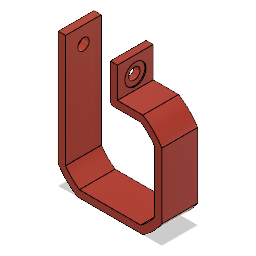
_extruder_mount.6a3fcada-6a02-4eac-834c-371bbe1a886d (Autodesk Fusion 360 design; units mm, degrees)
Autodesk Fusion 360 part; units mm, degrees
sketch "Sketch2" plane through (0, 0, 0) normal (0, 0, 1) x (1, 0, 0)
  line L0 (14.4655, -21) -> (-14.4655, -21)
  line L1 (-21, -14.4655) -> (-21, 14.4655)
  line L2 (1, 21) -> (14.4655, 21)
  line L3 (21, 14.4655) -> (21, -14.4655)
  line L4 (18.0312, -18.0312) -> (-18.0312, 18.0312) construction
  line L5 (-18.0312, -18.0312) -> (18.0312, 18.0312) construction
  arc A0 (21, 14.4655) -> (14.4655, 21) centre (0, 0) ccw
  arc A1 (-21, -14.4655) -> (-14.4655, -21) centre (0, 0) ccw
  arc A2 (14.4655, -21) -> (21, -14.4655) centre (0, 0) ccw
  line L6 (-21, 14.4655) -> (-21, 21)
  line L7 (0.0943, 21.9057) -> (0.0943, 41)
  line L8 (0.0943, 41) -> (-21, 41)
  line L9 (-21, 41) -> (-21, 21)
  line L10 (0.0943, 21.9057) -> (1, 21)
  line L11 (-24.5, 38.866) -> (-24.5, 21)
  line L12 (-24.5, 14.4655) -> (-24.5, 21)
  line L13 (-24.5, -15.5161) -> (-24.5, 14.4655)
  arc A3 (-24.5, -15.5161) -> (-15.5161, -24.5) centre (0, 0) ccw
  line L14 (15.5161, -24.5) -> (-15.5161, -24.5)
  arc A4 (15.5161, -24.5) -> (24.5, -15.5161) centre (0, 0) ccw
  line L15 (24.5, 15.5161) -> (24.5, -15.5161)
  arc A5 (24.5, 15.5161) -> (15.5161, 24.5) centre (0, 0) ccw
  line L16 (3.5, 24.5) -> (15.5161, 24.5)
  line L17 (3.5, 24.5) -> (3.5, 38.9603)
  line L18 (-24.5, 38.866) -> (-21, 38.866)
  line L19 (0.0943, 38.9603) -> (3.5, 38.9603)
  dimension "d3" = 51
  dimension "d6" = 20
  constraint perpendicular L0 L1
  constraint parallel L0 L2
  constraint parallel L1 L3
  constraint horizontal L0
  constraint coincident L4 A0.centre
  constraint coincident L5 A0.centre
  constraint coincident A0.centre A1.centre
  constraint coincident L4.end A1
  constraint concentric A0 A1
  constraint concentric A1 A2
  constraint coincident A0 L5.end
  constraint coincident A2 L4.start
  constraint coincident A1 L5.start
  constraint parallel L1 L6
  constraint vertical L7
  constraint horizontal L8
  constraint vertical L9
  constraint coincident L9 L18.end
  constraint perpendicular L9 L18
  constraint coincident L7 L19.start
  constraint perpendicular L17 L19
  constraint parallel L9 L11
  constraint parallel L6 L12
  constraint parallel L1 L13
  constraint concentric A1 A3
  constraint parallel L0 L14
  constraint concentric A2 A4
  constraint parallel L3 L15
  constraint concentric A0 A5
  constraint parallel L2 L16
  constraint parallel L7 L17
  measures "d3" diameter of A1
  measures "d6" distance of L6.end L8.end
extrude "Extrude9" add sketch "Sketch2" along normal blind 17 contours L0 L1 L2 L3 A0 A1 A2 L6 L7 L9 L10 L11 L12 L13 A3 L14 A4 L15 A5 L16 L17 L18 L19
sketch "Sketch7" plane through (-24.5, 0, 0) normal (-1, 0, 0) x (0, 0, 1)
  line L0 (0, 38.866) -> (0, -15.5161)
  line L1 (0, -15.5161) -> (17, -15.5161)
  line L2 (17, -15.5161) -> (17, 38.866)
  line L3 (17, 38.866) -> (0, 38.866)
sketch "Sketch8" plane through (3.5, 0, 0) normal (1, 0, 0) x (0, 0, -1)
  line L0 (0, 24.5) -> (0, 38.9603)
  line L1 (0, 38.9603) -> (-17, 38.9603)
  line L2 (-17, 38.9603) -> (-17, 24.5)
  line L3 (-17, 24.5) -> (0, 24.5)
  circle A0 centre (-8.5, 31) radius 2.7
  dimension "d32" = 5.4
  measures "d32" diameter of A0
extrude "Extrude10" cut sketch "Sketch8" against normal blind 50 contours A0
sketch "Sketch9" plane through (3.5, 0, 0) normal (1, 0, 0) x (0, 0, -1)
  circle A0 centre (-8.5, 31) radius 2.7
  line L0 (0, 24.5) -> (0, 38.9603)
  line L1 (0, 38.9603) -> (-17, 38.9603)
  line L2 (-17, 38.9603) -> (-17, 24.5)
  line L3 (-17, 24.5) -> (0, 24.5)
  circle A1 centre (-8.5, 31) radius 5
  dimension "d35" = 10
  constraint concentric A0 A1
  measures "d35" diameter of A1
extrude "Extrude11" cut sketch "Sketch9" against normal blind 0.5 contours A1
